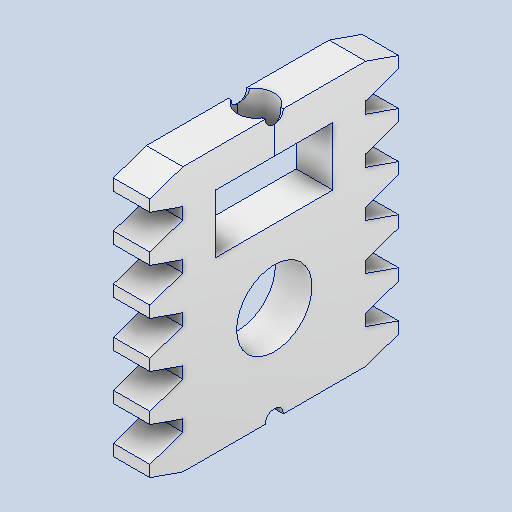
# Autodesk Inventor part: hand-grab-v5-Plate-2
Saved by Autodesk Inventor 2025.2 (Build 292293000, 293)
## iProperties
Created: 2025-05-11
Part Number: hand-grab-v5-Plate-2
Material: アルミニウム 6061
Document SubType Name: Modeling
Designer: haruy
Density: 2.7 g/cm^3
Appearance: アルミニウム - フラット
Author: haruy
Autodesk Inventor part; units mm, degrees
ref_plane "YZ Plane" through (0, 0, 0) normal (1, 0, 0) x (0, 1, 0)
ref_plane "XZ Plane" through (0, 0, 0) normal (0, 1, 0) x (-1, 0, 0)
ref_plane "XY Plane" through (0, 0, 0) normal (0, 0, 1) x (1, 0, 0)
derived "hand-grab-v5-Sketch-Base.ipt"
sketch "スケッチ1" plane through (0, 0, 0) normal (1, 0, 0) x (0, 1, 0)
  circle A0 centre (0, 0) radius 113.5 construction
  line L0 (196.3075, 10) -> (258.3075, 10)
  line L1 (258.3075, 10) -> (258.3075, -10)
  line L2 (258.3075, -10) -> (196.3075, -10)
  line L3 (196.3075, -10) -> (196.3075, 10)
  line L4 (196.3075, 5) -> (188.3075, 5)
  line L5 (188.3075, 5) -> (188.3075, -5)
  line L6 (188.3075, -5) -> (196.3075, -5)
  line L7 (196.3075, -5) -> (196.3075, 5)
  line L8 (188.3075, 2.5) -> (168.3075, 2.5)
  line L9 (168.3075, 2.5) -> (168.3075, -2.5)
  line L10 (168.3075, -2.5) -> (188.3075, -2.5)
  line L11 (188.3075, -2.5) -> (188.3075, 2.5)
  line L12 (183.3075, 2.5) -> (183.3075, -2.5)
  line L13 (183.3075, 4.619) -> (179.3075, 4.619)
  line L14 (179.3075, 4.619) -> (179.3075, -4.619)
  line L15 (179.3075, -4.619) -> (183.3075, -4.619)
  line L16 (183.3075, -4.619) -> (183.3075, 4.619)
  circle A1 centre (0, 0) radius 128.5 construction
  line L17 (290.4898, -280) -> (-352.5984, -280)
  circle A2 centre (151.819, -40) radius 25
  line L18 (0, 0) -> (-111.2843, -64.25) construction
  line L19 (0, 0) -> (-128.5, 0)
  line L20 (-111.724, -20) -> (-126.934, -20)
  circle A3 centre (151.819, -40) radius 10
  line L21 (68.4811, -90.5129) -> (145.7854, -32.0253)
  line L22 (157.4464, -48.2663) -> (72.3121, -106.2224)
  line L23 (0, 0) -> (0, -280)
  circle A4 centre (151.819, -40) radius 250.6731
  line L24 (151.819, -40) -> (-98.2939, -56.75)
  line L25 (151.819, -40) -> (0, -113.5)
  line L26 (151.819, -40) -> (-46.1675, -193.7477)
  line L27 (179.3075, 17) -> (142.3945, 17)
  line L28 (142.3945, 17) -> (142.3945, -12.5)
  line L29 (142.3945, -12.5) -> (179.3075, -12.5)
  line L30 (179.3075, -12.5) -> (179.3075, 17)
  line L31 (174.3075, 2.5) -> (174.3075, -2.5)
  line L32 (174.3075, 5) -> (170.3075, 5)
  line L33 (170.3075, 5) -> (170.3075, -5)
  line L34 (170.3075, -5) -> (174.3075, -5)
  line L35 (174.3075, -5) -> (174.3075, 5)
  line L36 (166.3075, 8) -> (174.3075, 8)
  line L37 (174.3075, 8) -> (174.3075, -8)
  line L38 (174.3075, -8) -> (166.3075, -8)
  line L39 (166.3075, -8) -> (166.3075, 8)
  line L40 (179.3075, -12.5) -> (142.3945, -12.5)
  line L41 (142.3945, -12.5) -> (142.3945, -17)
  line L42 (142.3945, -17) -> (179.3075, -17)
  line L43 (179.3075, -17) -> (179.3075, -12.5)
  line L44 (144.7515, -17) -> (143.1795, -12.5)
  line L45 (143.1795, -12.5) -> (141.6095, -12.5)
  line L46 (141.6095, -12.5) -> (140.0375, -17)
  line L47 (140.0375, -17) -> (144.7515, -17)
  line L48 (149.4625, -12.5) -> (147.8925, -12.5)
  line L49 (151.0345, -17) -> (149.4625, -12.5)
  line L50 (147.8925, -12.5) -> (146.3205, -17)
  line L51 (146.3205, -17) -> (151.0345, -17)
  line L52 (155.7455, -12.5) -> (154.1755, -12.5)
  line L53 (157.3175, -17) -> (155.7455, -12.5)
  line L54 (154.1755, -12.5) -> (152.6035, -17)
  line L55 (152.6035, -17) -> (157.3175, -17)
  line L56 (162.0285, -12.5) -> (160.4585, -12.5)
  line L57 (163.6005, -17) -> (162.0285, -12.5)
  line L58 (160.4585, -12.5) -> (158.8865, -17)
  line L59 (158.8865, -17) -> (163.6005, -17)
  line L60 (168.3115, -12.5) -> (166.7415, -12.5)
  line L61 (169.8835, -17) -> (168.3115, -12.5)
  line L62 (166.7415, -12.5) -> (165.1695, -17)
  line L63 (165.1695, -17) -> (169.8835, -17)
  line L64 (174.5945, -12.5) -> (173.0245, -12.5)
  line L65 (176.1665, -17) -> (174.5945, -12.5)
  line L66 (173.0245, -12.5) -> (171.4525, -17)
  line L67 (171.4525, -17) -> (176.1665, -17)
  line L68 (151.0345, -17) -> (152.6035, -17)
  line L69 (143.1795, -12.5) -> (143.1795, 28.2865)
  line L70 (171.4525, -17) -> (169.8835, -17)
  line L71 (180.8775, -12.5) -> (179.3075, -12.5)
  line L72 (182.4495, -17) -> (180.8775, -12.5)
  line L73 (179.3075, -12.5) -> (177.7355, -17)
  line L74 (177.7355, -17) -> (182.4495, -17)
  line L75 (179.3075, -15) -> (142.3945, -15)
  circle A5 centre (151.819, -40) radius 27
  line L76 (113.5, 148.4359) -> (113.5, -215.0589)
  arc A6 (-98.2939, -56.75) -> (68.4811, -90.5129) centre (0, 0) ccw
  arc A7 (-111.2843, -64.25) -> (72.3121, -106.2224) centre (0, 0) ccw
  line L77 (-98.2939, -56.75) -> (-111.2843, -64.25)
  line L78 (119.5722, -122.5175) -> (142.1536, -37.4348)
  line L79 (161.3299, -43.0891) -> (131.9849, -133.4377)
  arc A8 (-49.0169, -199.5899) -> (119.5722, -122.5175) centre (3.5876, -91.7346) ccw
  line L80 (-49.0169, -199.5899) -> (-55.5925, -213.0718)
  circle A9 centre (3.5876, -91.7346) radius 135 construction
  arc A10 (-55.5925, -213.0718) -> (131.9849, -133.4377) centre (3.5876, -91.7346) ccw
  line L81 (191.3075, 72) -> (196.3075, 72)
  line L82 (196.3075, 72) -> (196.3075, -72)
  line L83 (196.3075, -72) -> (191.3075, -72)
  line L84 (191.3075, -72) -> (191.3075, 72)
  line L85 (196.3075, -72) -> (156.819, -72)
  line L86 (156.819, -72) -> (156.819, -77)
  line L87 (156.819, -77) -> (196.3075, -77)
  line L88 (196.3075, -77) -> (196.3075, -72)
  line L89 (143.1795, 0) -> (179.3075, 0)
  circle A11 centre (151.819, -40) radius 8.25 construction
  circle A12 centre (151.819, -40) radius 13.25
  line L90 (156.819, -72) -> (140.7102, -47.2221)
  line L91 (144.8498, -28.7309) -> (191.3075, 0)
  circle A13 centre (193.8075, 0) radius 1.5
  circle A14 centre (193.8075, -36) radius 1.5
  line L92 (144.8498, 28.7309) -> (191.3075, 0)
  circle A15 centre (193.8075, 36) radius 1.5
  line L93 (196.3075, 72) -> (156.819, 72)
  line L94 (156.819, 72) -> (140.7102, 47.2221)
  circle A16 centre (151.819, 40) radius 13.25
  circle A17 centre (151.819, 40) radius 7.5
  circle A18 centre (151.819, -40) radius 7.5
  line L95 (151.819, -40) -> (151.819, -179.6263)
  circle A19 centre (156.3075, 0) radius 5.15
  circle A20 centre (141.3075, 0) radius 5.15
  circle A21 centre (141.3075, 0) radius 10.15
  line L96 (138.7877, 42.3976) -> (131.325, 1.8366)
  line L97 (138.7877, -42.3976) -> (131.325, -1.8366)
  circle A22 centre (143.1795, 0) radius 1.25
  circle A23 centre (179.3075, 0) radius 1.25
  circle A24 centre (-91.2843, -104.25) radius 4
  line L98 (-111.2843, -64.25) -> (-95.0076, -105.7117)
  circle A25 centre (91.2843, -104.25) radius 4
  line L99 (157.4464, -48.2663) -> (94.0062, -107.181)
  circle A26 centre (91.2843, -104.25) radius 1.5
  circle A27 centre (-91.2843, -104.25) radius 1.5
  line L100 (36, 107.6394) -> (36, 0)
  line L101 (36, 107.6394) -> (0, 107.6394)
  line L102 (0, 107.6394) -> (0, 0)
  circle A28 centre (0, 0) radius 120 construction
  circle A29 centre (0, -128.5) radius 4
  line L103 (1.027, -132.3659) -> (92.3113, -108.1159)
  line L104 (-1.027, -132.3659) -> (-92.3113, -108.1159)
  circle A30 centre (0, -128.5) radius 1.5
  point P0 (188.3075, 0)
  point P1 (142.3945, -12.5)
  point P2 (151.819, -17)
  point P3 (151.819, -17)
  point P4 (170.668, -17)
  point P5 (183.5696, -15)
  point P6 (174.3075, 0)
  point P7 (153.2871, -15.0431)
  point P8 (151.819, -15)
  point P9 (150.3509, -15.0431)
  point P10 (166.3075, 0)
  point P11 (150.3358, -15)
  point P12 (153.3021, -15)
  point P13 (179.3075, 0)
  point P14 (174.3075, 0)
  point P15 (151.819, -52.0973)
  point P16 (143.1795, 1.25)
  point P17 (143.1795, -1.25)
  point P18 (179.3075, 1.25)
  point P19 (179.3075, -1.25)
  dimension "d8" = 2.5
  dimension "d11" = 2.5
  measures "d8" diameter of A22
  measures "d11" diameter of A23
extrude "押し出し1" add sketch "スケッチ1" against normal blind 5 contours L91 L29 L69 A21 A19 L89 L39 L38 L37 L35 L10 L14 L30 | L30 L29 L91 | L10 L31 L89 A23 L14 | L73 L75 L65 L29 | L91 L61 L29 | L29 L66 L75 L61 L91 | A23 L89 L14 | L73 L42 L65 L75 | L62 L75 L57 L29 | L66 L42 L61 L75 | L69 A20 L89 A19 A21 | L42 L91 A5 L62 | A5 L91 L62 | L62 L91 A5 L57 L75 | L69 A22 L89 A20 | L29 L50 A5 L44 | A21 L89 A19 | A19 L89 A21 | L42 L57 A5 L91 | L58 A5 L53 L29 | L69 L89 A22 | A5 L50 L75 L44 | L58 L42 L53 A2 | A2 L53 L75 L58 | L58 L75 L53 A5 | L29 L54 A5 L49 | L75 L50 A2 L44 | A2 L50 L42 L44 | A5 L54 L75 L49 | L54 L42 L49 A2 | A2 L75 L54 | L75 A2 L49 picked at (178.4846, -0.0927) picked at (143.9796, -7.9935) picked at (143.5414, -3.4212) picked at (158.0756, -0.4056) picked at (151.265, -0.1598) picked at (143.9611, -0.2735)
mirror "ミラー1" about plane through (0, 143.1795, 0) normal (0, 0, 1) of "押し出し1"
sketch "スケッチ2" plane through (-5, 179.3075, -12.5) normal (0, 1, 0) x (1, 0, 0)
  circle A0 centre (2.5, -12.5) radius 2.5
  line L0 (5, -25) -> (0, -25) projected
  line L1 (2.5, -25) -> (2.5, 0)
  line L2 (5, 0) -> (0, 0) projected
  line L3 (5, -12.5) -> (0, -12.5)
  line L4 (0, 0) -> (0, -25) projected
  dimension "d3" = 5
  dimension "d4" = 0
  dimension "d5" = 0
  constraints: 4 end point, 3 midpoint, 1 centre point
  measures "d3" diameter of A0
  measures "d4" distance from line of A0.centre L1
  measures "d5" distance from line of L3 A0.centre
extrude "押し出し2" cut sketch "スケッチ2" against normal blind 5 contours L3 L1 A0 | A0 L1 L3 | L1 L3 A0 | A0 L3 L1
extrude "押し出し3" cut sketch "スケッチ1" against normal blind 10 contours L14 L89 A23 | A23 L89 L14 | A21 L89 A19 | A19 L89 A21 | A21 L89 A19 | A19 L89 A21 | A22 L89 L69 | L69 L89 A22
